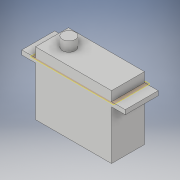
# Autodesk Inventor part: AssaultReaper500Servo
Saved by Autodesk Inventor 2018 (Build 220112000, 112)
## iProperties
Created: 2019-06-13
Part Number: AssaultReaper500Servo
Material: Generic
Document SubType Name: Modeling
Designer: anirudh
Density: 1 g/cm^3
Appearance: Default
Author: anirudh
Autodesk Inventor part; units mm, degrees
ref_plane "YZ Plane" through (0, 0, 0) normal (1, 0, 0) x (0, 1, 0)
ref_plane "XZ Plane" through (0, 0, 0) normal (0, 1, 0) x (-1, 0, 0)
ref_plane "XY Plane" through (0, 0, 0) normal (0, 0, 1) x (1, 0, 0)
sketch "Sketch1" plane through (0, 0, 0) normal (0, 1, 0) x (-1, 0, 0)
  line L0 (0, 0) -> (35.179, 0)
  line L1 (35.179, 0) -> (35.179, -15.24)
  line L2 (35.179, -15.24) -> (0, -15.24)
  line L3 (0, -15.24) -> (0, 0)
  dimension "d0" = 35.179
  dimension "d1" = 15.24
  constraints: 8 end point, 2 parallel, 1 horizontal, 1 perpendicular
  measures "d0" distance of L1.end L2.end
  measures "d1" distance of L0.end L1.end
extrude "Extrusion1" add sketch "Sketch1" along normal blind 29.21
ref_plane "Work Plane1" through (0, 24.765, 0) normal (0, 1, 0) x (1, 0, 0)
sketch "Sketch2" plane through (0, 24.765, 0) normal (0, 1, 0) x (1, 0, 0)
  line L0 (0, 0) -> (6.35, 0)
  line L1 (6.35, 0) -> (6.35, 15.24)
  line L2 (6.35, 15.24) -> (0, 15.24)
  line L3 (0, 15.24) -> (0, 0)
  line L4 (-35.179, 0) -> (0, 0) projected
  line L5 (-35.179, 0) -> (-41.529, 0)
  line L6 (-41.529, 0) -> (-41.529, 15.24)
  line L7 (-41.529, 15.24) -> (-35.179, 15.24)
  line L8 (-35.179, 15.24) -> (-35.179, 0)
  dimension "d5" = 6.35
  dimension "d6" = 6.35
  constraints: 16 end point, 4 parallel, 2 horizontal, 2 perpendicular, 1 point on line
  measures "d5" distance of L2.end L1.end
  measures "d6" distance of L6.end L7.end
extrude "Extrusion2" add sketch "Sketch2" against normal blind 2.032
sketch "Sketch3" plane through (0, 29.21, 0) normal (0, 1, 0) x (1, 0, 0)
  circle A0 centre (-27.3494, 7.62) radius 2.9655
  point P0 (0, 0)
  point P1 (-41.529, 0)
  point P2 (-41.529, 15.24)
  dimension "d10" = 5.9309
  constraints: 1 centre point
  measures "d10" diameter of A0
extrude "Extrusion3" add sketch "Sketch3" along normal blind 4.5212
body "Solid1"
